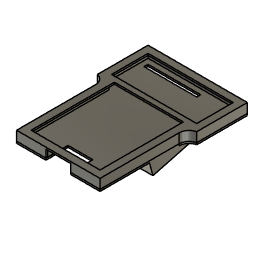
IO Stand v5 (Autodesk Fusion 360 design; units mm, degrees)
Autodesk Fusion 360 part; units mm, degrees
sketch "Sketch1" plane through (0, 0, 0) normal (0, 0, 1) x (1, 0, 0)
  line L0 (0, 0) -> (69.1, 0) construction
  line L1 (69.1, 0) -> (69.1, 77.1) construction
  line L2 (69.1, 77.1) -> (0, 77.1) construction
  line L3 (0, 77.1) -> (0, 0) construction
  line L4 (-1.6, -1.6) -> (70.7, -1.6)
  line L5 (70.7, -1.6) -> (70.7, 78.7)
  line L6 (70.7, 78.7) -> (-1.6, 78.7)
  line L7 (-1.6, 78.7) -> (-1.6, -1.6)
  line L8 (-3.2, 78.7) -> (72.3, 78.7)
  line L9 (72.3, 78.7) -> (72.3, -3.2)
  line L10 (72.3, -3.2) -> (-3.2, -3.2)
  line L11 (-3.2, -3.2) -> (-3.2, 78.7)
  line L12 (3.4, 73.7) -> (3.4, 3.4)
  line L13 (3.4, 3.4) -> (65.7, 3.4)
  line L14 (65.7, 3.4) -> (65.7, 73.7)
  line L15 (65.7, 73.7) -> (3.4, 73.7) construction
  line L16 (65.7, 73.7) -> (65.7, 78.7)
  line L17 (3.4, 73.7) -> (3.4, 78.7)
  line L18 (-5.55, 118.1) -> (74.65, 118.1)
  line L19 (74.65, 118.1) -> (74.65, 81.9)
  line L20 (74.65, 81.9) -> (-5.55, 81.9)
  line L21 (-5.55, 81.9) -> (-5.55, 118.1)
  line L22 (77.85, 78.7) -> (-8.75, 78.7)
  line L23 (-8.75, 78.7) -> (-8.75, 121.3)
  line L24 (-8.75, 121.3) -> (77.85, 121.3)
  line L25 (77.85, 121.3) -> (77.85, 78.7)
  line L26 (69.1, 77.1) -> (77.85, 77.1)
  line L27 (77.85, 77.1) -> (77.85, 78.7)
  line L28 (0, 77.1) -> (-8.75, 77.1)
  line L29 (-8.75, 77.1) -> (-8.75, 78.7)
  line L30 (77.85, 77.1) -> (79.45, 77.1)
  line L31 (79.45, 77.1) -> (79.45, 122.9)
  line L32 (79.45, 122.9) -> (77.85, 122.9)
  line L33 (77.85, 122.9) -> (77.85, 77.1)
  line L34 (-8.75, 77.1) -> (-10.35, 77.1)
  line L35 (-10.35, 77.1) -> (-10.35, 122.9)
  line L36 (-10.35, 122.9) -> (-8.75, 122.9)
  line L37 (-8.75, 122.9) -> (-8.75, 77.1)
  line L38 (-3.95, 116.5) -> (73.05, 116.5)
  line L39 (73.05, 116.5) -> (73.05, 83.5)
  line L40 (73.05, 83.5) -> (-3.95, 83.5)
  line L41 (-3.95, 83.5) -> (-3.95, 116.5)
  line L42 (-5.55, 118.1) -> (43.65, 118.1)
  line L43 (43.65, 118.1) -> (43.65, 112.9)
  line L44 (43.65, 112.9) -> (-5.55, 112.9)
  line L45 (-5.55, 112.9) -> (-5.55, 118.1)
  line L46 (23.35, -1.6) -> (45.75, -1.6)
  line L47 (45.75, -1.6) -> (45.75, -3.2)
  line L48 (45.75, -3.2) -> (23.35, -3.2)
  line L49 (23.35, -3.2) -> (23.35, -1.6)
  line L50 (-8.75, 122.9) -> (77.85, 122.9)
  line L51 (23.35, -1.6) -> (45.75, -1.6)
  line L52 (45.75, -1.6) -> (45.75, 16.8)
  line L53 (45.75, 16.8) -> (23.35, 16.8)
  line L54 (23.35, 16.8) -> (23.35, -1.6)
  point P0 (34.55, 77.1)
  point P1 (34.55, 118.1)
  point P2 (34.55, -1.6)
  dimension "d1" = 77.1
  dimension "d2" = 69.1
  dimension "d4" = 1.6
  dimension "d6" = 1.6
  dimension "d7" = 1.6
  dimension "d8" = 1.6
  dimension "d15" = -3.4
  dimension "d23" = 80.2
  dimension "d24" = 36.2
  dimension "d25" = -3.2
  dimension "d29" = 1.6
  dimension "d30" = 1.6
  dimension "d31" = 1.6
  dimension "d32" = 5.2
  dimension "d33" = 49.2
  dimension "d34" = 22.4
  dimension "d47" = 1.6
  dimension "d48" = 20
  constraint horizontal L0
  constraint vertical L1
  constraint horizontal L2
  constraint vertical L3
  constraint coincident L0.start L3.end
  constraint horizontal L8
  constraint vertical L9
  constraint horizontal L10
  constraint vertical L11
  constraint collinear L6 L8
  constraint midpoint L2 P0
  constraint coincident L6 L16.end
  constraint coincident L8 L16.end
  constraint coincident L8 L17.end
  constraint vertical L17
  constraint vertical L16
  constraint horizontal L18
  constraint vertical L19
  constraint horizontal L20
  constraint vertical L21
  constraint midpoint L18 P1
  constraint vertical P0 P1
  constraint collinear L8 L22
  constraint perpendicular L9 L26
  constraint perpendicular L3 L28
  constraint vertical L29
  constraint vertical L27
  constraint horizontal L30
  constraint vertical L31
  constraint horizontal L32
  constraint vertical L33
  constraint horizontal L34
  constraint vertical L35
  constraint horizontal L36
  constraint vertical L37
  constraint horizontal L42
  constraint vertical L43
  constraint horizontal L44
  constraint vertical L45
  constraint horizontal L46
  constraint vertical L47
  constraint horizontal L48
  constraint vertical L49
  constraint midpoint L46 P2
  constraint vertical P0 P2
  constraint coincident L4 L46.start
  constraint coincident L10 L47.end
  constraint horizontal L50
  constraint coincident L36.end L37.start
  constraint coincident L32.end L33.start
  constraint horizontal L51
  constraint vertical L52
  constraint horizontal L53
  constraint vertical L54
  constraint coincident L46.end L47.start
  measures "d1" distance of L0.end L1.end
  measures "d2" distance of L1.end L2.end
  measures "d6" distance of L7 L11
  measures "d7" distance of L5 L9
  measures "d8" distance of L4 L10
  measures "d23" distance of L18.start L18.end
  measures "d24" distance of L18.start L20.end
  measures "d29" distance of L35.end L36.end
  measures "d30" distance of L31.end L32.end
  measures "d32" distance of L42.end L43.end
  measures "d33" distance of L43.end L44.end
  measures "d34" distance of L46.start L46.end
  measures "d47" distance of L24 L50
  measures "d48" distance of L10 L53
extrude "Extrude1" add sketch "Sketch1" along normal blind 10.2 contours L4 L6 L7 L8 L12 L13 L17 L22 L54 | L4 L7 L10 L11 L28 L49 | L4 L13 L46 L51 L52 L54 | L4 L10 L46 L47 L48 L49 L51 | L7 L8 L11 L22 L28 | L4 L5 L6 L8 L13 L14 L16 L22 L52 | L4 L5 L9 L10 L26 L47 | L13 L52 L53 L54 | L6 L8 L12 L13 L14 L16 L17 L22 L52 L53 L54 | L6 L8 L22 L23 L24 L25 L33 L37 | L11 L22 L28 L29 L37 | L23 L29 L34 L35 L36 L37 | L5 L8 L9 L22 L26 | L9 L22 L26 L27 L33 | L24 L33 L37 L50 | L25 L27 L30 L31 L32 L33 | L18 L21 L38 L41 L42 L43 L44 L45 | L18 L19 L20 L21 L38 L39 L40 L41 L43 L44 | L38 L39 L40 L41 L43 L44 makes body 1
extrude "Extrude2" cut sketch "Sketch1" along normal up to surface (8.6 mm away) from surface at 1.6 contours L13 L52 L53 L54 | L6 L8 L12 L13 L14 L16 L17 L22 L52 L53 L54 | L38 L39 L40 L41 L43 L44 bodies 1
extrude "Extrude3" cut sketch "Sketch1" along normal blind 7 from surface at 1.6 contours L4 L6 L7 L8 L12 L13 L17 L22 L54 | L4 L13 L46 L51 L52 L54 | L4 L10 L46 L47 L48 L49 L51 | L4 L5 L6 L8 L13 L14 L16 L22 L52 | L6 L8 L22 L23 L24 L25 L33 L37 | L18 L21 L38 L41 L42 L43 L44 L45 | L18 L19 L20 L21 L38 L39 L40 L41 L43 L44 bodies 1
extrude "Extrude6" cut sketch "Sketch1" along normal up to surface (1.6 mm away) contours L4 L13 L46 L51 L52 L54 | L4 L10 L46 L47 L48 L49 L51 | L13 L52 L53 L54 bodies 1
fillet "Fillet1" radius 9 2 edges at (72.3, 77.1, 5.1) (-3.2, 77.1, 5.1) on bodies 1
ref_plane "WorkPlane2" through (34.55, 59.05, 1.6) normal (0, 0, 1) x (1, 0, 0)
split "Split2" by plane through (34.55, 59.05, 1.6) normal (0, 0, 1) bodies 1 makes body 2 at (1.2, 50.1307, 10.2)
sketch "Sketch2" plane through (0, 0, 0) normal (1, 0, 0) x (0, 1, 0)
  line L0 (77.1, 0) -> (0, 0)
  line L1 (41.55, 0) -> (44.6558, -11.5911)
  line L2 (44.6558, -11.5911) -> (87.9144, 0)
  line L3 (-3.2, 0) -> (78.7, 0)
  line L4 (87.9144, 0) -> (41.55, 0)
  point P0 (77.1, 0)
  point P1 (38.55, 0)
  point P2 (41.55, 0)
  dimension "d38" = 3
  dimension "d39" = 75
  dimension "d40" = 12
  constraint midpoint L0 P1
  constraint coincident L0 P2
  constraint coincident P2 L1.start
  constraint coincident L0 L2.end
  constraint perpendicular L1 L2
  measures "d38" distance of P1 P2
  measures "d39" angle of L1 L3
  measures "d40" distance of P2 L1.end
extrude "Extrude4" add sketch "Sketch2" along normal up to surface (26.55 mm away) from surface at -3.2 bodies 1
extrude "Extrude5" add 1 faces at (23.35, 58.0401, -3.8637) along direction (1, 0, 0) up to surface (26.55 mm away) from surface at 22.4 on bodies 1 bodies 1
ref_plane "WorkPlane1" through (34.55, 59.85, 5.1) normal (0, 0, -1) x (-1, 0, 0)
split "Split1" [suppressed]
equation "Clearance = 0.4 mm"
equation "WallThickness = 1.6 mm"
equation "d6 = WallThickness"
equation "d7 = WallThickness"
equation "d8 = WallThickness"
equation "d13 = 7 mm + WallThickness * 2"
equation "d15 = -5 mm + WallThickness"
equation "d18 = WallThickness"
equation "d25 = -WallThickness * 2"
equation "WallHeight = 10 mm"
equation "d29 = WallThickness"
equation "d30 = WallThickness"
equation "d31 = WallThickness"
equation "d32 = 4.8 mm + Clearance"
equation "d33 = 48.8 mm + Clearance"
equation "d34 = 22 mm + Clearance"
equation "d47 = WallThickness"
equation "d48 = BeltCutoutLength"
equation "BeltCutoutLength = 20 mm"
